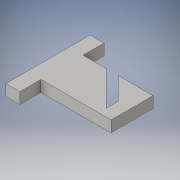
# Autodesk Inventor part: connector
Saved by Autodesk Inventor 2016 (Build 200138000, 138)
## iProperties
Created: 2015-12-05
Part Number: connector
Material: Generic
Document SubType Name: Modeling
Designer: acd
Density: 1 g/cm^3
Appearance: Default
Author: acd
Autodesk Inventor part; units mm, degrees
ref_plane "YZ Plane" through (0, 0, 0) normal (1, 0, 0) x (0, 1, 0)
ref_plane "XZ Plane" through (0, 0, 0) normal (0, 1, 0) x (-1, 0, 0)
ref_plane "XY Plane" through (0, 0, 0) normal (0, 0, 1) x (1, 0, 0)
sketch "Sketch1" plane through (0, 0, 0) normal (0, 1, 0) x (-1, 0, 0)
  line L0 (5, 30) -> (-5, 30)
  line L1 (-5, 30) -> (-5, 15)
  line L2 (-5, 15) -> (-55, 15)
  line L3 (-55, 15) -> (-55, -15)
  line L4 (-55, -15) -> (-30, -15)
  line L5 (-30, -15) -> (-46.0981, 1.0981)
  line L6 (-46.0981, 1.0981) -> (-46.0981, 9.5833)
  line L7 (-46.0981, 9.5833) -> (-21.5147, -15)
  line L8 (-21.5147, -15) -> (-5, -15)
  line L9 (-5, -15) -> (-5, -30)
  line L10 (-5, -30) -> (5, -30)
  line L11 (5, -30) -> (5, 30)
  point P0 (0, 0)
  constraints: 24 end point, 7 perpendicular, 3 parallel, 1 horizontal
sketch "Sketch2" plane through (0, 0, 0) normal (0, 1, 0) x (-1, 0, 0)
  point P0 (0, 0)
extrude "Extrusion1" add sketch "Sketch1" along normal blind 8
body "Solid1"
